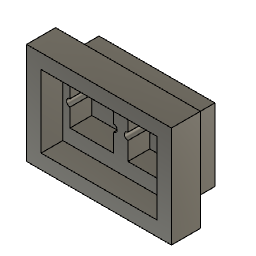
buttonboxbase v7 (Autodesk Fusion 360 design; units mm, degrees)
Autodesk Fusion 360 part; units mm, degrees
note: some values were not read from the file. Set by a fixed rule: which sketch regions a step uses.
sketch "Sketch1" plane through (0, 0, 0) normal (0, 1, 0) x (1, 0, 0)
  line L0 (7, -3.5) -> (-7, -3.5)
  line L1 (-7, -3.5) -> (-7, 3.5)
  line L2 (-7, 3.5) -> (7, 3.5)
  line L3 (7, 3.5) -> (7, -3.5)
  line L4 (7, -3.5) -> (-7, 3.5) construction
  line L5 (-7, -3.5) -> (7, 3.5) construction
  circle A0 centre (-6, 0) radius 0.5
  circle A1 centre (-1, 0) radius 0.5
  circle A2 centre (1, 0) radius 0.5
  circle A3 centre (6, 0) radius 0.5
  dimension "d3" = 14
  dimension "d4" = 7
  dimension "d7" = 1
  dimension "d8" = 1
  dimension "d9" = 1
  dimension "d10" = 1
  constraint horizontal L0
  constraint perpendicular L0 L1
  constraint parallel L0 L2
  constraint parallel L1 L3
  constraint coincident L4 origin
  constraint coincident L5 origin
  measures "d3" distance of L1.end L2.end
  measures "d4" distance of L0.end L1.end
  measures "d7" diameter of A0
  measures "d8" diameter of A1
  measures "d9" diameter of A2
  measures "d10" diameter of A3
sketch "Sketch2" plane through (0, 0, 0) normal (0, -1, 0) x (1, 0, 0)
  circle A0 centre (-1, 0) radius 0.5
  circle A1 centre (1, 0) radius 0.5
  circle A2 centre (6, 0) radius 0.5
  circle A3 centre (-6, 0) radius 0.5
  line L0 (-7, -3.5) -> (7, -3.5)
  line L1 (7, -3.5) -> (7, 3.5)
  line L2 (7, 3.5) -> (-7, 3.5)
  line L3 (-7, 3.5) -> (-7, -3.5)
  line L4 (-6, 2.5) -> (-6, -2.5)
  line L5 (6, -2.5) -> (6, 2.5)
  line L6 (6, -2.5) -> (1, -2.5)
  line L7 (1, -2.5) -> (1, 2.5)
  line L8 (1, 2.5) -> (6, 2.5)
  line L9 (-6, -2.5) -> (-6, 2.5)
  line L10 (-6, 2.5) -> (-1, 2.5)
  line L11 (-1, 2.5) -> (-1, -2.5)
  line L12 (-1, -2.5) -> (-6, -2.5)
  constraint parallel L3 L4
  constraint parallel L1 L5
  constraint perpendicular L4 L10
  constraint perpendicular L10 L11
sketch "Sketch3" plane through (0, 0, 0) normal (0, -1, 0) x (1, 0, 0)
sketch "Sketch4" plane through (0, 0, 0) normal (0, 1, 0) x (1, 0, 0)
  line L0 (-8, -5) -> (8, -5)
  line L1 (8, -5) -> (8, 5)
  line L2 (8, 5) -> (-8, 5)
  line L3 (-8, 5) -> (-8, -5)
  line L4 (-8, -5) -> (8, 5) construction
  line L5 (8, -5) -> (-8, 5) construction
  line L6 (-1, 0) -> (-1, -3)
  line L7 (-1, -3) -> (-7, -3)
  line L8 (-7, -3) -> (-7, 3)
  line L9 (-7, 3) -> (-1, 3)
  line L10 (-1, 3) -> (-1, 0)
  line L11 (1, 3) -> (1, -3)
  line L12 (1, -3) -> (7, -3)
  line L13 (7, -3) -> (7, 3)
  line L14 (7, 3) -> (1, 3)
  dimension "d16" = 16
  dimension "d17" = 10
  constraint horizontal L0
  constraint perpendicular L0 L1
  constraint parallel L0 L2
  constraint parallel L1 L3
  constraint coincident L4 origin
  constraint coincident L5 origin
  constraint perpendicular L6 L7
  constraint perpendicular L7 L8
  constraint perpendicular L8 L9
  constraint perpendicular L11 L12
  constraint perpendicular L12 L13
  constraint perpendicular L11 L14
  measures "d16" distance of L1.end L2.end
  measures "d17" distance of L0.end L1.end
sketch "Sketch5" plane through (0, 0, 0) normal (0, -1, 0) x (1, 0, 0)
  line L0 (-8, 5) -> (-8, -5)
  line L1 (-8, -5) -> (8, -5)
  line L2 (8, -5) -> (8, 5)
  line L3 (8, 5) -> (-8, 5)
  line L4 (-1, -3) -> (-1, 3)
  line L5 (-1, 3) -> (-7, 3)
  line L6 (-7, 3) -> (-7, -3)
  line L7 (-7, -3) -> (-1, -3)
  line L8 (1, -3) -> (1, 3)
  line L9 (1, 3) -> (7, 3)
  line L10 (7, 3) -> (7, -3)
  line L11 (7, -3) -> (1, -3)
  constraint perpendicular L4 L5
  constraint perpendicular L5 L6
  constraint perpendicular L4 L7
  constraint perpendicular L8 L9
  constraint perpendicular L9 L10
  constraint perpendicular L8 L11
sketch "Sketch6" plane through (0, 0, 0) normal (0, -1, 0) x (1, 0, 0)
  line L0 (-1, 3) -> (-1, -3)
  line L1 (-1, -3) -> (-7, -3)
  line L2 (-7, -3) -> (-7, 3)
  line L3 (-7, 3) -> (-1, 3)
  line L4 (1, 3) -> (7, 3)
  line L5 (7, 3) -> (7, -3)
  line L6 (7, -3) -> (1, -3)
  line L7 (1, -3) -> (1, 3)
  line L8 (-8, 5) -> (-8, -5)
  line L9 (-8, -5) -> (8, -5)
  line L10 (8, -5) -> (8, 5)
  line L11 (8, 5) -> (-8, 5)
  circle A0 centre (-7, 0) radius 0.25
  circle A1 centre (-1, 0) radius 0.25
  circle A2 centre (1, 0) radius 0.25
  circle A3 centre (7, 0) radius 0.25
  dimension "d23" = 0.5
  dimension "d24" = 0.5
  dimension "d25" = 0.5
  dimension "d26" = 0.5
  constraint midpoint L2 A0.centre
  constraint midpoint L0 A1.centre
  constraint midpoint L7 A2.centre
  constraint midpoint L5 A3.centre
  measures "d23" diameter of A0
  measures "d24" diameter of A1
  measures "d25" diameter of A2
  measures "d26" diameter of A3
sketch "Sketch7" plane through (0, 4, 0) normal (0, 1, 0) x (-1, 0, 0)
  circle A0 centre (1, 0) radius 0.25
  circle A1 centre (-1, 0) radius 0.25
  circle A2 centre (7, 0) radius 0.25
  circle A3 centre (-7, 0) radius 0.25
  line L0 (8, -5) -> (8, 5)
  line L1 (8, 5) -> (-8, 5)
  line L2 (-8, 5) -> (-8, -5)
  line L3 (-8, -5) -> (8, -5)
  line L4 (-10, -7) -> (10, -7)
  line L5 (10, -7) -> (10, 7)
  line L6 (10, 7) -> (-10, 7)
  line L7 (-10, 7) -> (-10, -7)
  circle A4 centre (-7, 0) radius 0.25
  circle A5 centre (-1, 0) radius 0.25
  circle A6 centre (1, 0) radius 0.25
  circle A7 centre (7, 0) radius 0.25
  dimension "d29" = 2
  constraint concentric A3 A4
  constraint concentric A1 A5
  constraint concentric A0 A6
  constraint concentric A2 A7
sketch "Sketch8" plane through (0, 0, 0) normal (0, -1, 0) x (1, 0, 0)
  line L0 (-8, 5) -> (-8, -5)
  line L1 (-8, -5) -> (8, -5)
  line L2 (8, -5) -> (8, 5)
  line L3 (8, 5) -> (-8, 5)
  arc A0 (1, 0.25) -> (1, -0.25) centre (1, 0) ccw
  line L4 (1, 0.25) -> (1, 3)
  line L5 (1, 3) -> (7, 3)
  line L6 (7, 3) -> (7, 0.25)
  arc A1 (7, -0.25) -> (7, 0.25) centre (7, 0) ccw
  line L7 (7, -0.25) -> (7, -3)
  line L8 (7, -3) -> (1, -3)
  line L9 (1, -3) -> (1, -0.25)
  arc A2 (-1, -0.25) -> (-1, 0.25) centre (-1, 0) ccw
  line L10 (-1, -0.25) -> (-1, -3)
  line L11 (-1, -3) -> (-7, -3)
  line L12 (-7, -3) -> (-7, -0.25)
  arc A3 (-7, 0.25) -> (-7, -0.25) centre (-7, 0) ccw
  line L13 (-7, 0.25) -> (-7, 3)
  line L14 (-7, 3) -> (-1, 3)
  line L15 (-1, 3) -> (-1, 0.25)
  circle A4 centre (-6.5, 4) radius 0.5
  circle A5 centre (-6.5, -4) radius 0.5
  circle A6 centre (6.5, -4) radius 0.5
  circle A7 centre (6.5, 4) radius 0.5
ref_plane "WorkPlane1" through (0, -6, 0) normal (0, -1, 0) x (-1, 0, 0)
sketch "Sketch11" plane through (0, 0, 0) normal (0, -1, 0) x (1, 0, 0)
sketch "Sketch12" plane through (0, 4, 0) normal (0, 1, 0) x (-1, 0, 0)
  circle A0 centre (1, 0) radius 0.25
  circle A1 centre (-1, 0) radius 0.25
  circle A2 centre (7, 0) radius 0.25
  circle A3 centre (-7, 0) radius 0.25
  line L0 (-11, -8) -> (11, -8)
  line L1 (11, -8) -> (11, 8)
  line L2 (11, 8) -> (-11, 8)
  line L3 (-11, 8) -> (-11, -8)
sketch "Sketch13" plane through (0, 0, 0) normal (0, -1, 0) x (1, 0, 0)
sketch "Sketch14" plane through (0, 0, 0) normal (0, -1, 0) x (1, 0, 0)
sketch "Sketch15" plane through (0, 0, 0) normal (0, 1, 0) x (1, 0, 0)
  line L0 (8, -5) -> (-8, -5)
  line L1 (-8, -5) -> (-8, 5)
  line L2 (-8, 5) -> (8, 5)
  line L3 (8, 5) -> (8, -5)
  line L4 (8, -5) -> (-8, 5) construction
  line L5 (-8, -5) -> (8, 5) construction
  dimension "d43" = 16
  dimension "d44" = 10
  constraint horizontal L0
  constraint perpendicular L0 L1
  constraint parallel L0 L2
  constraint parallel L1 L3
  constraint coincident L4 origin
  constraint coincident L5 origin
  measures "d43" distance of L1.end L2.end
  measures "d44" distance of L0.end L1.end
extrude "Extrude9" add sketch "Sketch15" along normal blind 5
sketch "Sketch16" plane through (0, 0, 0) normal (0, -1, 0) x (1, 0, 0)
  line L0 (-8, -5) -> (8, -5)
  line L1 (8, -5) -> (8, 5)
  line L2 (8, 5) -> (-8, 5)
  line L3 (-8, 5) -> (-8, -5)
  line L4 (7, 3) -> (1, 3)
  line L5 (1, 3) -> (1, -3)
  line L6 (1, -3) -> (7, -3)
  line L7 (7, -3) -> (7, 3)
  line L8 (7, 3) -> (1, -3) construction
  line L9 (1, 3) -> (7, -3) construction
  line L10 (-1, 0) -> (-4, 0)
  line L11 (-1, 0) -> (-1, 3)
  line L12 (-1, 0) -> (-1, -3)
  line L13 (-1, -3) -> (-7, -3)
  line L14 (-7, -3) -> (-7, 3)
  line L15 (-7, 3) -> (-1, 3)
  point P0 (4, 0)
  dimension "d48" = 6
  dimension "d49" = 6
  dimension "d50" = 1
  dimension "d51" = 3
  dimension "d52" = 3
  dimension "d53" = 6
  dimension "d54" = 6
  constraint horizontal L4
  constraint perpendicular L4 L5
  constraint parallel L4 L6
  constraint parallel L5 L7
  constraint coincident L8 P0
  constraint coincident L9 P0
  constraint perpendicular L5 L13
  constraint perpendicular L13 L14
  measures "d48" distance of L5.end L6.end
  measures "d49" distance of L4.end L5.end
  measures "d50" distance of origin L10.start
  measures "d51" distance of L10.start L10.end
  measures "d52" distance of L10.start L11.end
  measures "d53" distance of L12.end L13.end
  measures "d54" distance of L13.end L14.end
extrude "Extrude10" cut sketch "Sketch16" against normal blind 3 contours L4 L5 L6 L7 | L11 L12 L13 L14 L15
sketch "Sketch17" plane through (0, 0, 0) normal (0, -1, 0) x (1, 0, 0)
  line L0 (-7, 3) -> (-1, 3)
  line L1 (-1, 3) -> (-1, -3)
  line L2 (-1, -3) -> (-7, -3)
  line L3 (-7, -3) -> (-7, 3)
  line L4 (1, 3) -> (7, 3)
  line L5 (7, 3) -> (7, -3)
  line L6 (7, -3) -> (1, -3)
  line L7 (1, -3) -> (1, 3)
  line L8 (-8, -5) -> (8, -5)
  line L9 (8, -5) -> (8, 5)
  line L10 (8, 5) -> (-8, 5)
  line L11 (-8, 5) -> (-8, -5)
  line L12 (-10, -7) -> (10, -7)
  line L13 (10, -7) -> (10, 7)
  line L14 (10, 7) -> (-10, 7)
  line L15 (-10, 7) -> (-10, -7)
  dimension "d57" = 2
extrude "Extrude11" add sketch "Sketch17" along normal blind 3 and the other way blind 1 contours L12 L13 L14 L15
sketch "Sketch18" plane through (0, 0, 0) normal (0, -1, 0) x (1, 0, 0)
  line L0 (-7, 3) -> (-1, 3)
  line L1 (-1, 3) -> (-1, -3)
  line L2 (-1, -3) -> (-7, -3)
  line L3 (-7, -3) -> (-7, 3)
  line L4 (1, 3) -> (7, 3)
  line L5 (7, 3) -> (7, -3)
  line L6 (7, -3) -> (1, -3)
  line L7 (1, -3) -> (1, 3)
  line L8 (-8, -5) -> (8, -5)
  line L9 (8, -5) -> (8, 5)
  line L10 (8, 5) -> (-8, 5)
  line L11 (-8, 5) -> (-8, -5)
  circle A0 centre (1, 0) radius 0.5
  circle A1 centre (7, 0) radius 0.5
  circle A2 centre (-1, 0) radius 0.5
  circle A3 centre (-7, 0) radius 0.5
  dimension "d62" = 1
  dimension "d63" = 1
  dimension "d64" = 1
  dimension "d65" = 1
  constraint midpoint L7 A0.centre
  constraint midpoint L5 A1.centre
  constraint midpoint L1 A2.centre
  constraint midpoint L3 A3.centre
  measures "d62" diameter of A0
  measures "d63" diameter of A1
  measures "d64" diameter of A2
  measures "d65" diameter of A3
extrude "Extrude12" cut sketch "Sketch18" against normal blind 5 contours L3 A3 | L3 A3 | L1 A2 | L1 A2 | L7 A0 | L7 A0 | L5 A1 | L5 A1
sketch "Sketch19" plane through (0, 0, 0) normal (0, -1, 0) x (1, 0, 0)
  line L0 (-8, -5) -> (8, -5)
  line L1 (8, 5) -> (-8, 5)
  line L2 (-8, 5) -> (-8, -5)
  arc A0 (1, 0.5) -> (1, -0.5) centre (1, 0) ccw
  arc A1 (7, -0.5) -> (7, 0.5) centre (7, 0) ccw
  line L3 (7, -3) -> (1, -3)
  line L4 (1, -3) -> (1, -0.5)
  arc A2 (-1, -0.5) -> (-1, 0.5) centre (-1, 0) ccw
  line L5 (-1, -0.5) -> (-1, -3)
  line L6 (-1, -3) -> (-7, -3)
  line L7 (-7, -3) -> (-7, -0.5)
  arc A3 (-7, 0.5) -> (-7, -0.5) centre (-7, 0) ccw
  line L8 (-7, 0.5) -> (-7, 3)
  line L9 (-7, 3) -> (-1, 3)
  line L10 (-8, 5) -> (8, 5)
  line L11 (8, 5) -> (8, -5)
  line L12 (8, -5) -> (-8, -5)
  line L13 (-8, -5) -> (-8, 5)
  constraint horizontal L10
  constraint vertical L11
  constraint horizontal L12
  constraint vertical L13
  constraint coincident L0.end L11.end
  constraint coincident L1.end L2.start
sketch "Sketch20" plane through (0, -10, 0) normal (0, 1, 0) x (-1, 0, 0)
  line L0 (-8, -5) -> (8, -5)
  line L1 (8, -5) -> (8, 5)
  line L2 (8, 5) -> (-8, 5)
  line L3 (-8, 5) -> (-8, -5)
  line L4 (-7, -4) -> (7, -4)
  line L5 (7, -4) -> (7, 4)
  line L6 (7, 4) -> (-7, 4)
  line L7 (-7, 4) -> (-7, -4)
  dimension "d73" = -1
sketch "Sketch21" plane through (0, -13, 0) normal (0, -1, 0) x (1, 0, 0)
  line L0 (-8, -5) -> (8, -5)
  line L1 (8, -5) -> (8, 5)
  line L2 (8, 5) -> (-8, 5)
  line L3 (-8, 5) -> (-8, -5)
  circle A0 centre (-4, 0) radius 2
  circle A1 centre (4, 0) radius 2
named bodies: "BoxBase"
